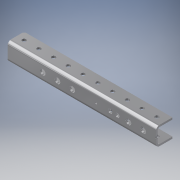
# Autodesk Inventor part: am-2222
Saved by Autodesk Inventor 2016 (Build 200138000, 138)
## iProperties
Category: Drive Base Kit
Company: Autodesk Inc.
Created: 2012-12-27
Part Number: am-2222
Material: Aluminum 6061
Document SubType Name: Modeling
Designer: Autodesk Inc.
Density: 1 g/cm^3
Catalog Web Link: www.andymark.com
Vendor: AndyMark Inc.
Appearance: Aluminum - Flat
Author: Autodesk Inc.
Autodesk Inventor part; units mm, degrees
ref_plane "YZ Plane" through (0, 0, 0) normal (1, 0, 0) x (0, 1, 0)
ref_plane "XZ Plane" through (0, 0, 0) normal (0, 1, 0) x (-1, 0, 0)
ref_plane "XY Plane" through (0, 0, 0) normal (0, 0, 1) x (1, 0, 0)
sketch "Sketch1" plane through (0, 0, 0) normal (0, 0, 1) x (1, 0, 0)
  line L0 (6.35, 28.575) -> (25.4, 28.575)
  line L1 (6.35, 31.75) -> (25.4, 31.75)
  line L2 (25.4, 0) -> (6.35, 0)
  arc A0 (0, 6.35) -> (6.35, 0) centre (6.35, 6.35) ccw
  line L3 (0, 6.35) -> (0, 25.4)
  arc A1 (6.35, 31.75) -> (0, 25.4) centre (6.35, 25.4) ccw
  line L4 (6.35, 31.75) -> (25.4, 31.75)
  line L5 (25.4, 28.575) -> (6.35, 28.575)
  arc A2 (6.35, 28.575) -> (3.175, 25.4) centre (6.35, 25.4) ccw
  line L6 (3.175, 25.4) -> (3.175, 6.35)
  arc A3 (3.175, 6.35) -> (6.35, 3.175) centre (6.35, 6.35) ccw
  line L7 (6.35, 3.175) -> (25.4, 3.175)
  line L8 (28.575, 3.175) -> (28.575, 0)
  line L9 (25.4, 31.75) -> (28.575, 31.75)
  line L10 (28.575, 28.575) -> (25.4, 28.575)
  line L11 (28.575, 31.75) -> (28.575, 28.575)
  line L12 (28.575, 0) -> (25.4, 0)
  line L13 (28.575, 3.175) -> (28.575, 0)
  line L14 (25.4, 3.175) -> (28.575, 3.175)
  point P0 (0, 0)
  constraints: 30 end point, 8 point on circle, 4 centre point
extrude "Extrusion1" add sketch "Sketch1" against normal blind 762
chamfer "Chamfer1" distance 3.175 angle 45 4 edges at (28.575, 30.1625, 0) (28.575, 1.5875, 0) (28.575, 30.1625, -762) (28.575, 1.5875, -762)
sketch "Sketch2" plane through (6.35, 31.75, 0) normal (0, 1, 0) x (1, 0, 0)
  line L0 (19.05, 0) -> (0, 0) projected
  line L1 (22.225, 3.175) -> (22.225, 758.825) projected
  point P0 (-6.35, 0)
  point P1 (9.525, 12.7)
  dimension "d5" = 12.7
  dimension "d6" = 12.7
  measures "d5" distance from line of point (9.525, 12.7) L0
  measures "d6" distance from line of point (9.525, 12.7) L1
hole "Hole1" at (15.875, 31.75, -12.7) direction (0, -1, 0) diameter 6.7056 end through all
pattern_linear "Rectangular Pattern1" count 30 spacing 25.4 along (0, 0, -1) of "Hole1"
sketch "Sketch3" plane through (0, 6.35, 0) normal (-1, 0, 0) x (0, 0, 1)
  line L0 (0, 19.05) -> (-762, 19.05)
  line L1 (-762, 19.05) -> (-762, 0)
  line L2 (0, 0) -> (-762, 0)
  line L3 (0, 0) -> (0, 19.05)
  circle A0 centre (-701.3194, 9.525) radius 4.8006
  circle A1 centre (-111.4298, 9.525) radius 4.8006
  circle A2 centre (-189.2808, 9.525) radius 3.683
  circle A3 centre (-278.1808, 9.525) radius 3.683
  circle A4 centre (-483.7938, 9.525) radius 3.683
  circle A5 centre (-572.6938, 9.525) radius 3.683
  circle A6 centre (-471.1065, 9.525) radius 3.683
  circle A7 centre (-585.4065, 9.525) radius 3.683
  circle A8 centre (-290.8935, 9.525) radius 3.683
  circle A9 centre (-176.5935, 9.525) radius 3.683
  circle A10 centre (-553.7327, 9.525) radius 4.8006
  circle A11 centre (-528.3327, 9.525) radius 4.8006
  circle A12 centre (-502.9327, 9.525) radius 4.8006
  circle A13 centre (-259.0673, 9.525) radius 4.8006
  circle A14 centre (-233.6673, 9.525) radius 4.8006
  circle A15 centre (-208.2673, 9.525) radius 4.8006
  circle A16 centre (-609.6, 9.525) radius 1.5875
  circle A17 centre (-152.4, 9.525) radius 1.5875
  circle A18 centre (-381, 5.969) radius 4.8006
  circle A19 centre (-86.0298, 9.525) radius 4.8006
  circle A20 centre (-675.9194, 9.525) radius 4.8006
  circle A21 centre (-650.5194, 9.525) radius 4.8006
  circle A22 centre (-60.6298, 9.525) radius 4.8006
  point P0 (0, -6.35)
  point P1 (-762, -6.35)
  constraints: 23 centre point, 8 end point
extrude "Extrusion2" cut sketch "Sketch3" against normal up to next contours A0 | A1 | A2 | A3 | A4 | A5 | A6 | A7 | A8 | A9 | A10 | A11 | A12 | A13 | A14 | A15 | A16 | A17 | A18 | A19 | A20 | A21 | A22
sketch "Sketch4" plane through (6.35, 31.75, 0) normal (0, 1, 0) x (1, 0, 0)
  line L0 (-21.9023, 506.5738) -> (102.4291, 506.5738)
  line L1 (102.4291, 506.5738) -> (102.4291, -101.978)
  line L2 (102.4291, -101.978) -> (-21.9023, -101.978)
  line L3 (-21.9023, -101.978) -> (-21.9023, 506.5738)
  point P0 (-6.35, 0)
  constraints: 8 end point, 2 parallel, 1 horizontal, 1 perpendicular
extrude "Extrusion3" cut sketch "Sketch4" against normal blind 50.8
body "Solid1"
